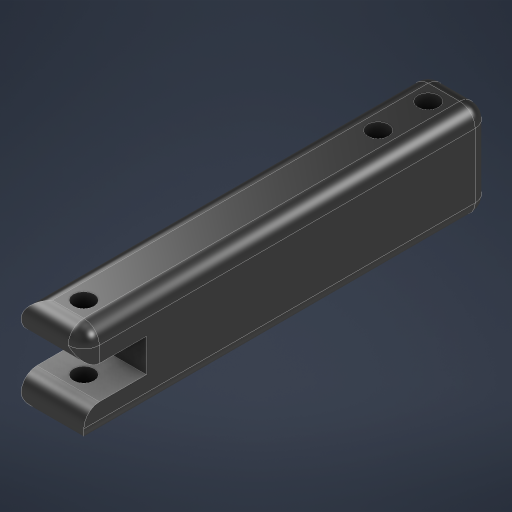
# Autodesk Inventor part: wing bar
Saved by Autodesk Inventor 2024 (Build 280153000, 153)
## iProperties
Created: 2023-12-24
Part Number: wing bar
Material: Generic
Document SubType Name: Modeling
Designer: elite
Density: 1 g/cm^3
Appearance: Glossy - Black
Author: elite
Autodesk Inventor part; units mm, degrees
ref_plane "YZ Plane" through (0, 0, 0) normal (1, 0, 0) x (0, 1, 0)
ref_plane "XZ Plane" through (0, 0, 0) normal (0, 1, 0) x (-1, 0, 0)
ref_plane "XY Plane" through (0, 0, 0) normal (0, 0, 1) x (1, 0, 0)
sketch "Sketch1" plane through (0, 0, 0) normal (1, 0, 0) x (0, 1, 0)
  line L0 (0, 0) -> (6.35, 0)
  line L1 (6.35, 0) -> (6.35, -12.7)
  line L2 (6.35, -12.7) -> (13.081, -12.7)
  line L3 (13.081, -12.7) -> (13.081, 0)
  line L4 (13.081, 0) -> (19.431, 0)
  line L5 (19.431, 0) -> (19.431, -82.55)
  line L6 (19.431, -82.55) -> (0, -82.55)
  line L7 (0, -82.55) -> (0, 0)
  dimension "d0" = 6.35
  dimension "d1" = 12.7
  dimension "d2" = 6.731
  dimension "d11" = 6.35
  dimension "d12" = 82.55
  dimension "d18" = 12.7
  constraints: 16 end point, 4 perpendicular, 2 horizontal, 2 vertical
  measures "d0" distance of L0.start L0.end
  measures "d1" distance of L0.end L1.end
  measures "d2" distance of L1.end L2.end
  measures "d11" distance of L3.end L4.end
  measures "d12" distance of L4.end L5.end
  measures "d18" distance of L2.end L3.end
extrude "Extrusion1" add sketch "Sketch1" along normal blind 12.7
sketch "Sketch3" plane through (0, 19.431, 0) normal (0, 1, 0) x (1, 0, 0)
  line L0 (0, 12.7) -> (12.7, 12.7) projected
  line L1 (12.7, 12.7) -> (0, 12.7)
  line L2 (0, 12.7) -> (0, 0)
  line L3 (0, 0) -> (12.7, 0)
  line L4 (12.7, 0) -> (12.7, 12.7)
  line L5 (0, 0) -> (12.7, 12.7)
  circle A0 centre (6.35, 6.35) radius 2.1082
  line L6 (0, 82.55) -> (12.7, 82.55) projected
  line L7 (6.35, 82.55) -> (6.35, 76.2)
  circle A1 centre (6.35, 76.2) radius 2.1082
  dimension "d13" = 4.2164
  dimension "d16" = 6.35
  dimension "d17" = 4.2164
  constraints: 12 end point, 2 centre point, 2 midpoint, 2 parallel, 1 coincident, 1 horizontal, 1 perpendicular, 1 vertical
  measures "d13" diameter of A0
  measures "d16" distance of L7.start L7.end
  measures "d17" diameter of A1
extrude "Extrusion3" cut sketch "Sketch3" against normal blind 28.575 contours A0 L5 | L5 A0 | A1
fillet "Fillet1" radius 3.175 1 edges at (12.7, 19.431, -41.275)
fillet "Fillet2" radius 3.175 14 edges at (11.7701, 18.5011, 0) (12.7, 14.6685, 0) (4.7625, 19.431, 0) (0, 19.431, -41.275) (11.7701, 18.5011, -82.55) (12.7, 8.128, -82.55) (4.7625, 19.431, -82.55) (0, 9.7155, -82.55) (12.7, 0, -41.275) (6.35, 0, -82.55) (0, 0, -41.275) (6.35, 0, 0) (6.35, 6.35, 0) (6.35, 13.081, 0)
sketch "Sketch5" plane through (3.175, 19.431, -3.175) normal (0, 1, 0) x (1, 0, 0)
  circle A0 centre (3.175, 73.025) radius 2.1082 projected
  line L0 (3.175, 73.025) -> (3.175, 62.865)
  circle A1 centre (3.175, 62.865) radius 2.1082
  point P0 (-3.175, -3.175)
  dimension "d26" = 10.16
  constraints: 2 end point, 1 centre point, 1 coincident, 1 vertical
  measures "d26" distance of L0.start L0.end
extrude "Extrusion5" cut sketch "Sketch5" against normal blind 25.4 contours A1
body "Solid1"
